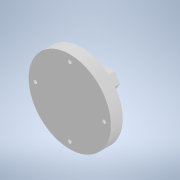
# Autodesk Inventor part: Exagono
Saved by Autodesk Inventor 2020.1 (Build 241239000, 239)
## iProperties
Created: 2019-12-03
Part Number: Exagono
Material: Generic
Document SubType Name: Modeling
Designer: Daniel
Density: 1 g/cm^3
Appearance: Default
Author: Daniel
Autodesk Inventor part; units mm, degrees
ref_plane "YZ Plane" through (0, 0, 0) normal (1, 0, 0) x (0, 1, 0)
ref_plane "XZ Plane" through (0, 0, 0) normal (0, 1, 0) x (-1, 0, 0)
ref_plane "XY Plane" through (0, 0, 0) normal (0, 0, 1) x (1, 0, 0)
sketch "Sketch1" plane through (0, 0, 0) normal (0, 0, 1) x (1, 0, 0)
  line L0 (-2, 3.4641) -> (2, 3.4641) projected
  line L1 (-4, 0) -> (-2, 3.4641) projected
  line L2 (-2, -3.4641) -> (-4, 0) projected
  line L3 (2, -3.4641) -> (-2, -3.4641) projected
  line L4 (4, 0) -> (2, -3.4641) projected
  line L5 (2, 3.4641) -> (4, 0) projected
  line L6 (-4, 0) -> (-2, 3.4641) projected
  line L7 (-2, 3.4641) -> (2, 3.4641) projected
  line L8 (2, 3.4641) -> (4, 0) projected
  line L9 (4, 0) -> (2, -3.4641) projected
  line L10 (2, -3.4641) -> (-2, -3.4641) projected
  line L11 (-2, -3.4641) -> (-4, 0) projected
  circle A0 centre (0, 0) radius 7.5 projected
  circle A1 centre (0, 0) radius 6.5
  point P0 (0, 0)
  dimension "d0" = 1
  constraints: 1 centre point
  measures "d0" radial gap between concentric circles of A0 A1
extrude "Extrusion1" add sketch "Sketch1" against normal blind 10 contours L0 L5 L4 L3 L2 L1
ref_plane "Work Plane2" through (0, 0, 0) normal (0, 0, 1) x (1, 0, 0)
sketch "Sketch3" plane through (0, 0, 0) normal (0, 0, 1) x (1, 0, 0)
  circle A0 centre (0, 0) radius 6.5 projected
  point P0 (0, 0)
extrude "Extrusion2" add sketch "Sketch3" along normal blind 2
sketch "Sketch4" plane through (0, 0, 2) normal (0, 0, 1) x (1, 0, 0)
  circle A0 centre (0, 0) radius 17.25
  circle A1 centre (0, 0) radius 14.45 construction
  point P0 (14.45, 0)
  point P1 (-14.45, 0)
  point P2 (0, 14.45)
  point P3 (0, -14.45)
  dimension "d5" = 34.5
  dimension "d6" = 28.9
  constraints: 4 point on circle, 2 centre point, 2 coincident
  measures "d5" diameter of A0
  measures "d6" diameter of A1
extrude "Extrusion3" add sketch "Sketch4" along normal blind 5
hole "Hole1" at (14.45, 0, 2) at (-14.45, 0, 2) at (0, 14.45, 2) at (0, -14.45, 2) direction (0, 0, 1) diameter 1.5 end through all
body "Solid1"
